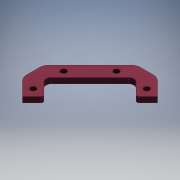
# Autodesk Inventor part: VAM_housing_bottom
Saved by Autodesk Inventor 2016 (Build 200138000, 138)
## iProperties
Created: 2015-12-08
Part Number: VAM_housing_bottom
Material: Generic
Document SubType Name: Modeling
Designer: lk8187
Density: 1 g/cm^3
Appearance: Smooth - Dark Maroon
Author: lk8187
Autodesk Inventor part; units mm, degrees
ref_plane "YZ Plane" through (0, 0, 0) normal (1, 0, 0) x (0, 1, 0)
ref_plane "XZ Plane" through (0, 0, 0) normal (0, 1, 0) x (-1, 0, 0)
ref_plane "XY Plane" through (0, 0, 0) normal (0, 0, 1) x (1, 0, 0)
derived "VAM_housing.ipt"
sketch "Sketch1" plane through (0, 0, 0) normal (0, 0, 1) x (1, 0, 0)
  line L0 (-2.1213, 22.6274) -> (-22.6274, 2.1213)
  line L1 (-22.6274, -2.1213) -> (-2.1213, -22.6274)
  line L2 (2.1213, -22.6274) -> (22.6274, -2.1213)
  line L3 (22.6274, 2.1213) -> (2.1213, 22.6274)
  arc A0 (2.1213, 22.6274) -> (-2.1213, 22.6274) centre (0, 20.5061) ccw
  arc A1 (22.6274, -2.1213) -> (22.6274, 2.1213) centre (20.5061, 0) ccw
  arc A2 (-2.1213, -22.6274) -> (2.1213, -22.6274) centre (0, -20.5061) ccw
  arc A3 (-22.6274, 2.1213) -> (-22.6274, -2.1213) centre (-20.5061, 0) ccw
  line L4 (-30.5, 5.5624) -> (-5.5624, 30.5)
  line L5 (-5.5624, 30.5) -> (5.5624, 30.5)
  line L6 (5.5624, 30.5) -> (30.5, 5.5624)
  line L7 (30.5, 5.5624) -> (30.5, -5.5624)
  line L8 (30.5, -5.5624) -> (5.5624, -30.5)
  line L9 (5.5624, -30.5) -> (-5.5624, -30.5)
  line L10 (-5.5624, -30.5) -> (-30.5, -5.5624)
  line L11 (-30.5, -5.5624) -> (-30.5, 5.5624)
  line L12 (8.1317, 22.2739) -> (22.2739, 8.1317) construction
  line L13 (22.2739, -8.1317) -> (8.1317, -22.2739) construction
  line L14 (-8.1317, -22.2739) -> (-22.2739, -8.1317) construction
  line L15 (-22.2739, 8.1317) -> (-8.1317, 22.2739) construction
  line L16 (12.3744, 12.3744) -> (18.0312, 18.0312) construction
  line L17 (12.3744, -12.3744) -> (18.0312, -18.0312) construction
  line L18 (-12.3744, -12.3744) -> (-18.0312, -18.0312) construction
  line L19 (-12.3744, 12.3744) -> (-18.0312, 18.0312) construction
  circle A4 centre (0, 0) radius 14
  circle A5 centre (0, 0) radius 9
  line L20 (14.4957, 21.5668) -> (8.8388, 15.9099)
  line L21 (-15.9099, -8.8388) -> (-21.5668, -14.4957)
  point P0 (0, 30.5)
  point P1 (0, -30.5)
  point P2 (30.5, 0)
  point P3 (-30.5, 0)
  point P4 (15.2028, 15.2028)
  point P5 (15.2028, -15.2028)
  point P6 (-15.2028, -15.2028)
  point P7 (-15.2028, 15.2028)
extrude "Extrusion1" add sketch "Sketch1" along normal blind 3 contours L0 A3 L1 L21 L10 L11 L4 L5 L6 L20 L3 A0
hole "Hole1" at (-8.1317, 22.2739, 0) at (8.1317, 22.2739, 0) at (22.2739, 8.1317, 0) at (22.2739, -8.1317, 0) at (8.1317, -22.2739, 0) at (-8.1317, -22.2739, 0) at (-22.2739, -8.1317, 0) at (-22.2739, 8.1317, 0) direction (0, 0, 1) diameter 3 end through all
fillet "Fillet1" radius 5 4 edges at (-30.5, 5.5624, 1.5) (-30.5, -5.5624, 1.5) (-5.5624, 30.5, 1.5) (5.5624, 30.5, 1.5)
fillet "Fillet2" radius 1 2 edges at (-15.9099, -8.8388, 1.5) (8.8388, 15.9099, 1.5)
body "Solid1"
